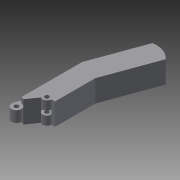
# Autodesk Inventor part: Finger_Upper_main_1
Saved by Autodesk Inventor 2015 (Build 190159000, 159)
## iProperties
Created: 2016-07-06
Part Number: Finger_Upper_main_1
Material: Generic
Document SubType Name: Modeling
Designer: Neelotpal Nag
Density: 1 g/cm^3
Appearance: Default
Author: Neelotpal Nag
Autodesk Inventor part; units mm, degrees
ref_plane "YZ Plane" through (0, 0, 0) normal (1, 0, 0) x (0, 1, 0)
ref_plane "XZ Plane" through (0, 0, 0) normal (0, 1, 0) x (-1, 0, 0)
ref_plane "XY Plane" through (0, 0, 0) normal (0, 0, 1) x (1, 0, 0)
sketch "Sketch1" plane through (0, 0, 0) normal (0, 0, 1) x (1, 0, 0)
  line L0 (0, 30) -> (8.5505, 53.4923)
  circle A0 centre (0, 0) radius 1
  circle A1 centre (0, 0) radius 2.25
  line L1 (0, 0) -> (2.25, 0) construction
  line L2 (0, 0) -> (0, 1)
  line L3 (0, 2.25) -> (0, 30)
  circle A2 centre (5.7358, 8.1915) radius 1
  circle A3 centre (5.7358, 8.1915) radius 2
  line L4 (0, 0) -> (0.5736, 0.8192)
  line L5 (1.2905, 1.8431) -> (4.5886, 6.5532)
  line L6 (5.7358, 8.1915) -> (4.7358, 8.1915)
  line L7 (3.7358, 8.1915) -> (0, 8.1915)
  line L8 (0, 30) -> (9.3969, 26.5798)
  line L9 (9.3969, 26.5798) -> (17.9474, 50.0721)
  line L10 (9.3969, 26.5798) -> (9.3969, 8.1915)
  line L11 (9.3969, 8.1915) -> (7.7358, 8.1915)
  arc A4 (17.9474, 50.0721) -> (8.5505, 53.4923) centre (10.287, 43.6442) ccw
  line L12 (0, 30) -> (9.3969, 26.5798)
  line L13 (9.3969, 26.5798) -> (17.9474, 50.0721)
  line L14 (0, 30) -> (8.5505, 53.4923)
  dimension "d7" = 2
  dimension "d0" = 30
  dimension "d1" = 25
  dimension "d3" = 2
  dimension "d4" = 4.5
  dimension "d5" = 10
  dimension "d8" = 4
  dimension "d11" = 10
  dimension "d16" = 10
  constraints: 30 end point, 10 point on circle, 7 coincident, 6 perpendicular, 4 centre point, 3 collinear, 3 vertical, 1 horizontal, 1 horizontal alignment, 1 point on line, 2 other
  measures "d0" distance of L2.start L0.start
  measures "d1" distance of L0.start L0.end
  measures "d3" diameter of A0
  measures "d4" diameter of A1
  measures "d5" distance of L1.start L6.start
  measures "d8" diameter of A3
  measures "d11" distance of L0.start L8.end
  measures "d16" radius of A4
extrude "Extrusion1" add sketch "Sketch1" along normal mid plane 10 contours L8 L10 L11 A3 L7 L3
extrude "Extrusion2" add sketch "Sketch1" along normal mid plane 10 contours L7 A3 L5 A1 L3
extrude "Extrusion3" add sketch "Sketch1" along normal mid plane 10 contours L0 A4 L9 L8
extrude "Extrusion4" add sketch "Sketch1" along normal mid plane 5 contours A1
sketch "Sketch2" plane through (0, 0, 2.5) normal (0, 0, 1) x (1, 0, 0)
  line L0 (0, 7.0508) -> (-2.1324, 0.718)
  arc A0 (0, 2.25) -> (1.2905, 1.8431) centre (0, 0) ccw projected
  line L1 (0, 7.0508) -> (0, 2.25)
  arc A1 (0, 2.25) -> (-2.1324, 0.718) centre (0, 0) ccw
  constraints: 4 end point, 3 point on circle, 1 centre point, 1 concentric, 1 tangent, 1 vertical
extrude "Extrusion5" add sketch "Sketch2" against normal blind 5
extrude "Extrusion6" add sketch "Sketch1" along normal mid plane 10 contours A3
extrude "Extrusion7" cut sketch "Sketch1" along normal mid plane 2 contours A3
body "Solid1"
